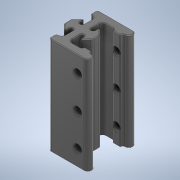
# Autodesk Inventor part: 80-20 Slider -  ( Length = 3 inch )
Saved by Autodesk Inventor 2020.2 (Build 242310000, 310)
## iProperties
Created: 2020-02-10
Part Number: 80-20 Slider -  ( Length = 3 inch )
Material: Generic
Document SubType Name: Modeling
Designer: lucas
Density: 1 g/cm^3
Appearance: Smooth - Black
Author: lucas
Autodesk Inventor part; units mm, degrees
ref_plane "YZ Plane" through (0, 0, 0) normal (1, 0, 0) x (0, 1, 0)
ref_plane "XZ Plane" through (0, 0, 0) normal (0, 1, 0) x (-1, 0, 0)
ref_plane "XY Plane" through (0, 0, 0) normal (0, 0, 1) x (1, 0, 0)
sketch "Sketch1" plane through (0, 0, 0) normal (0, 1, 0) x (-1, 0, 0)
  circle A0 centre (0, 0) radius 2.6035
  arc A1 (-12.6998, -10.5664) -> (-10.5664, -12.6998) centre (-10.5918, -10.5918) ccw
  arc A2 (-9.5504, -12.7) -> (-10.5664, -12.6998) centre (-10.0584, -12.7) ccw
  line L0 (-9.5504, -12.7) -> (-6.3331, -12.7)
  arc A3 (-5.3171, -12.7) -> (-6.3331, -12.7) centre (-5.8251, -12.7) ccw
  line L1 (-5.3171, -12.7) -> (-4.3434, -12.7)
  arc A4 (-4.3434, -12.7) -> (-4.3434, -10.4902) centre (-4.3434, -11.5951) ccw
  line L2 (-4.3434, -10.4902) -> (-6.4748, -10.4902)
  arc A5 (-7.1932, -8.7558) -> (-6.4748, -10.4902) centre (-6.4748, -9.4742) ccw
  line L3 (-7.1932, -8.7558) -> (-3.8632, -5.4257)
  arc A6 (-1.6181, -4.4958) -> (-3.8632, -5.4257) centre (-1.6181, -7.6708) ccw
  line L4 (-1.6181, -4.4958) -> (1.6181, -4.4958)
  arc A7 (3.8632, -5.4257) -> (1.6181, -4.4958) centre (1.6181, -7.6708) ccw
  line L5 (3.8632, -5.4257) -> (7.1932, -8.7558)
  arc A8 (6.4748, -10.4902) -> (7.1932, -8.7558) centre (6.4748, -9.4742) ccw
  line L6 (6.4748, -10.4902) -> (4.3434, -10.4902)
  arc A9 (4.3434, -10.4902) -> (4.3434, -12.7) centre (4.3434, -11.5951) ccw
  line L7 (4.3434, -12.7) -> (5.3171, -12.7)
  arc A10 (6.3331, -12.7) -> (5.3171, -12.7) centre (5.8251, -12.7) ccw
  line L8 (6.3331, -12.7) -> (9.5504, -12.7)
  arc A11 (10.5664, -12.6998) -> (9.5504, -12.7) centre (10.0584, -12.7) ccw
  arc A12 (10.5664, -12.6998) -> (12.6998, -10.5664) centre (10.5918, -10.5918) ccw
  arc A13 (12.7, -9.5504) -> (12.6998, -10.5664) centre (12.7, -10.0584) ccw
  line L9 (12.7, -9.5504) -> (12.7, -6.3331)
  arc A14 (12.7, -5.3171) -> (12.7, -6.3331) centre (12.7, -5.8251) ccw
  line L10 (12.7, -5.3171) -> (12.7, -4.3434)
  arc A15 (12.7, -4.3434) -> (10.4902, -4.3434) centre (11.5951, -4.3434) ccw
  line L11 (10.4902, -4.3434) -> (10.4902, -6.4748)
  arc A16 (8.7558, -7.1932) -> (10.4902, -6.4748) centre (9.4742, -6.4748) ccw
  line L12 (8.7558, -7.1932) -> (5.4257, -3.8632)
  arc A17 (4.4958, -1.6181) -> (5.4257, -3.8632) centre (7.6708, -1.6181) ccw
  line L13 (4.4958, -1.6181) -> (4.4958, 1.6181)
  arc A18 (5.4257, 3.8632) -> (4.4958, 1.6181) centre (7.6708, 1.6181) ccw
  line L14 (5.4257, 3.8632) -> (8.7558, 7.1932)
  arc A19 (10.4902, 6.4748) -> (8.7558, 7.1932) centre (9.4742, 6.4748) ccw
  line L15 (10.4902, 6.4748) -> (10.4902, 4.3434)
  arc A20 (10.4902, 4.3434) -> (12.7, 4.3434) centre (11.5951, 4.3434) ccw
  line L16 (12.7, 4.3434) -> (12.7, 5.3171)
  arc A21 (12.7, 6.3331) -> (12.7, 5.3171) centre (12.7, 5.8251) ccw
  line L17 (12.7, 6.3331) -> (12.7, 9.5504)
  arc A22 (12.6998, 10.5664) -> (12.7, 9.5504) centre (12.7, 10.0584) ccw
  arc A23 (12.6998, 10.5664) -> (10.5664, 12.6998) centre (10.5918, 10.5918) ccw
  arc A24 (9.5504, 12.7) -> (10.5664, 12.6998) centre (10.0584, 12.7) ccw
  line L18 (9.5504, 12.7) -> (6.3331, 12.7)
  arc A25 (5.3171, 12.7) -> (6.3331, 12.7) centre (5.8251, 12.7) ccw
  line L19 (5.3171, 12.7) -> (4.3434, 12.7)
  arc A26 (4.3434, 12.7) -> (4.3434, 10.4902) centre (4.3434, 11.5951) ccw
  line L20 (4.3434, 10.4902) -> (6.4748, 10.4902)
  arc A27 (7.1932, 8.7558) -> (6.4748, 10.4902) centre (6.4748, 9.4742) ccw
  line L21 (7.1932, 8.7558) -> (3.8632, 5.4257)
  arc A28 (1.6181, 4.4958) -> (3.8632, 5.4257) centre (1.6181, 7.6708) ccw
  line L22 (1.6181, 4.4958) -> (-1.6181, 4.4958)
  arc A29 (-3.8632, 5.4257) -> (-1.6181, 4.4958) centre (-1.6181, 7.6708) ccw
  line L23 (-3.8632, 5.4257) -> (-7.1932, 8.7558)
  arc A30 (-6.4748, 10.4902) -> (-7.1932, 8.7558) centre (-6.4748, 9.4742) ccw
  line L24 (-6.4748, 10.4902) -> (-4.3434, 10.4902)
  arc A31 (-4.3434, 10.4902) -> (-4.3434, 12.7) centre (-4.3434, 11.5951) ccw
  line L25 (-4.3434, 12.7) -> (-5.3171, 12.7)
  arc A32 (-6.3331, 12.7) -> (-5.3171, 12.7) centre (-5.8251, 12.7) ccw
  line L26 (-6.3331, 12.7) -> (-9.5504, 12.7)
  arc A33 (-10.5664, 12.6998) -> (-9.5504, 12.7) centre (-10.0584, 12.7) ccw
  arc A34 (-10.5664, 12.6998) -> (-12.6998, 10.5664) centre (-10.5918, 10.5918) ccw
  arc A35 (-12.7, 9.5504) -> (-12.6998, 10.5664) centre (-12.7, 10.0584) ccw
  line L27 (-12.7, 9.5504) -> (-12.7, 6.3331)
  arc A36 (-12.7, 5.3171) -> (-12.7, 6.3331) centre (-12.7, 5.8251) ccw
  line L28 (-12.7, 5.3171) -> (-12.7, 4.3434)
  arc A37 (-12.7, 4.3434) -> (-10.4902, 4.3434) centre (-11.5951, 4.3434) ccw
  line L29 (-10.4902, 4.3434) -> (-10.4902, 6.4748)
  arc A38 (-8.7558, 7.1932) -> (-10.4902, 6.4748) centre (-9.4742, 6.4748) ccw
  line L30 (-8.7558, 7.1932) -> (-5.4257, 3.8632)
  arc A39 (-4.4958, 1.6181) -> (-5.4257, 3.8632) centre (-7.6708, 1.6181) ccw
  line L31 (-4.4958, 1.6181) -> (-4.4958, -1.6181)
  arc A40 (-5.4257, -3.8632) -> (-4.4958, -1.6181) centre (-7.6708, -1.6181) ccw
  line L32 (-5.4257, -3.8632) -> (-8.7558, -7.1932)
  arc A41 (-10.4902, -6.4748) -> (-8.7558, -7.1932) centre (-9.4742, -6.4748) ccw
  line L33 (-10.4902, -6.4748) -> (-10.4902, -4.3434)
  arc A42 (-10.4902, -4.3434) -> (-12.7, -4.3434) centre (-11.5951, -4.3434) ccw
  line L34 (-12.7, -4.3434) -> (-12.7, -5.3171)
  arc A43 (-12.7, -6.3331) -> (-12.7, -5.3171) centre (-12.7, -5.8251) ccw
  line L35 (-12.7, -6.3331) -> (-12.7, -9.5504)
  arc A44 (-12.6998, -10.5664) -> (-12.7, -9.5504) centre (-12.7, -10.0584) ccw
  arc A45 (-10.1902, -6.4748) -> (-8.9679, -6.9811) centre (-9.4742, -6.4748) ccw
  arc A46 (-8.9679, 6.9811) -> (-10.1902, 6.4748) centre (-9.4742, 6.4748) ccw
  line L36 (-8.9679, 6.9811) -> (-5.6379, 3.651)
  arc A47 (-4.7958, 1.6181) -> (-5.6379, 3.651) centre (-7.6708, 1.6181) ccw
  arc A48 (-5.6379, -3.651) -> (-4.7958, -1.6181) centre (-7.6708, -1.6181) ccw
  line L37 (-4.7958, 1.6181) -> (-4.7958, -1.6181)
  line L38 (-5.6379, -3.651) -> (-8.9679, -6.9811)
  line L39 (-10.1902, 6.4748) -> (-10.1902, 4.3434)
  line L40 (-10.1902, -6.4748) -> (-10.1902, -4.3434)
  line L41 (-13.7, 19.05) -> (-39.37, 19.05)
  line L42 (-13, -4.3434) -> (-13, -10.5918)
  line L43 (-13.7, -19.05) -> (-39.37, -19.05)
  line L44 (-3.005, 15.2109) -> (-3.005, 14.9109)
  arc A49 (-13, 4.3434) -> (-10.1902, 4.3434) centre (-11.5951, 4.3434) ccw
  line L45 (-13, 4.3434) -> (-13, 10.5918)
  arc A50 (-10.1902, -4.3434) -> (-13, -4.3434) centre (-11.5951, -4.3434) ccw
  line L46 (-39.37, 19.05) -> (-39.37, -19.05)
  line L47 (-13.7, 19.05) -> (-8.89, 19.05)
  line L48 (-8.89, 19.05) -> (-8.89, 13)
  line L49 (-8.89, 13) -> (-10.5918, 13)
  line L50 (-13.7, -19.05) -> (-8.89, -19.05)
  line L51 (-8.89, -19.05) -> (-8.89, -13)
  line L52 (-8.89, -13) -> (-10.5918, -13)
  arc A51 (-10.5918, 13) -> (-13, 10.5918) centre (-10.5918, 10.5918) ccw
  arc A52 (-13, -10.5918) -> (-10.5918, -13) centre (-10.5918, -10.5918) ccw
  line L53 (-15.875, -23.3068) -> (-15.875, 30.5551) construction
  line L54 (-35.6132, -5.4257) -> (-38.9432, -8.7558)
  line L55 (-38.2248, -10.4902) -> (-36.0934, -10.4902)
  line L56 (-36.0934, -12.7) -> (-37.0671, -12.7)
  arc A53 (-36.0934, -12.7) -> (-36.0934, -10.4902) centre (-36.0934, -11.5951) ccw
  arc A54 (-37.1757, -3.8632) -> (-36.2458, -1.6181) centre (-39.4208, -1.6181) ccw
  arc A55 (-33.3681, -4.4958) -> (-35.6132, -5.4257) centre (-33.3681, -7.6708) ccw
  line L57 (-30.1319, -4.4958) -> (-33.3681, -4.4958)
  arc A56 (-37.0671, -12.7) -> (-38.0831, -12.7) centre (-37.5751, -12.7) ccw
  arc A57 (-36.2458, 1.6181) -> (-37.1757, 3.8632) centre (-39.4208, 1.6181) ccw
  line L58 (-36.2458, -1.6181) -> (-36.2458, 1.6181)
  arc A58 (-24.5568, 8.7558) -> (-25.2752, 10.4902) centre (-25.2752, 9.4742) ccw
  arc A59 (-19.0502, 10.5664) -> (-19.05, 9.5504) centre (-19.05, 10.0584) ccw
  arc A60 (-19.0502, 10.5664) -> (-21.1836, 12.6998) centre (-21.1582, 10.5918) ccw
  arc A61 (-22.1996, 12.7) -> (-21.1836, 12.6998) centre (-21.6916, 12.7) ccw
  line L59 (-25.2752, 10.4902) -> (-27.4066, 10.4902)
  line L60 (-25.4169, 12.7) -> (-22.1996, 12.7)
  arc A62 (-26.4329, 12.7) -> (-25.4169, 12.7) centre (-25.9249, 12.7) ccw
  arc A63 (-27.4066, 12.7) -> (-27.4066, 10.4902) centre (-27.4066, 11.5951) ccw
  line L61 (-27.4066, 12.7) -> (-26.4329, 12.7)
  arc A64 (-22.9942, -7.1932) -> (-21.2598, -6.4748) centre (-22.2758, -6.4748) ccw
  line L62 (-24.5568, -8.7558) -> (-27.8868, -5.4257)
  line L63 (-19.05, -6.3331) -> (-19.05, -9.5504)
  arc A65 (-25.2752, -10.4902) -> (-24.5568, -8.7558) centre (-25.2752, -9.4742) ccw
  arc A66 (-19.05, -9.5504) -> (-19.0502, -10.5664) centre (-19.05, -10.0584) ccw
  line L64 (-27.4066, -10.4902) -> (-25.2752, -10.4902)
  arc A67 (-21.1836, -12.6998) -> (-19.0502, -10.5664) centre (-21.1582, -10.5918) ccw
  arc A68 (-21.1836, -12.6998) -> (-22.1996, -12.7) centre (-21.6916, -12.7) ccw
  line L65 (-22.1996, -12.7) -> (-25.4169, -12.7)
  arc A69 (-25.4169, -12.7) -> (-26.4329, -12.7) centre (-25.9249, -12.7) ccw
  arc A70 (-27.4066, -10.4902) -> (-27.4066, -12.7) centre (-27.4066, -11.5951) ccw
  line L66 (-26.4329, -12.7) -> (-27.4066, -12.7)
  arc A71 (-38.9432, -8.7558) -> (-38.2248, -10.4902) centre (-38.2248, -9.4742) ccw
  line L67 (-40.5058, -7.1932) -> (-37.1757, -3.8632)
  line L68 (-38.0831, -12.7) -> (-41.3004, -12.7)
  arc A72 (-42.2402, -6.4748) -> (-40.5058, -7.1932) centre (-41.2242, -6.4748) ccw
  arc A73 (-41.3004, -12.7) -> (-42.3164, -12.6998) centre (-41.8084, -12.7) ccw
  line L69 (-42.2402, -4.3434) -> (-42.2402, -6.4748)
  arc A74 (-42.2402, -4.3434) -> (-44.45, -4.3434) centre (-43.3451, -4.3434) ccw
  line L70 (-44.45, -5.3171) -> (-44.45, -4.3434)
  arc A75 (-44.45, -6.3331) -> (-44.45, -5.3171) centre (-44.45, -5.8251) ccw
  line L71 (-44.45, -9.5504) -> (-44.45, -6.3331)
  arc A76 (-44.4498, -10.5664) -> (-44.45, -9.5504) centre (-44.45, -10.0584) ccw
  arc A77 (-44.4498, -10.5664) -> (-42.3164, -12.6998) centre (-42.3418, -10.5918) ccw
  line L72 (-37.1757, 3.8632) -> (-40.5058, 7.1932)
  line L73 (-42.2402, 6.4748) -> (-42.2402, 4.3434)
  arc A78 (-44.45, 4.3434) -> (-42.2402, 4.3434) centre (-43.3451, 4.3434) ccw
  line L74 (-38.9432, 8.7558) -> (-35.6132, 5.4257)
  line L75 (-44.45, 4.3434) -> (-44.45, 5.3171)
  arc A79 (-40.5058, 7.1932) -> (-42.2402, 6.4748) centre (-41.2242, 6.4748) ccw
  line L76 (-36.0934, 10.4902) -> (-38.2248, 10.4902)
  arc A80 (-44.45, 5.3171) -> (-44.45, 6.3331) centre (-44.45, 5.8251) ccw
  line L77 (-44.45, 6.3331) -> (-44.45, 9.5504)
  arc A81 (-44.45, 9.5504) -> (-44.4498, 10.5664) centre (-44.45, 10.0584) ccw
  arc A82 (-38.2248, 10.4902) -> (-38.9432, 8.7558) centre (-38.2248, 9.4742) ccw
  arc A83 (-36.0934, 10.4902) -> (-36.0934, 12.7) centre (-36.0934, 11.5951) ccw
  line L78 (-37.0671, 12.7) -> (-36.0934, 12.7)
  arc A84 (-38.0831, 12.7) -> (-37.0671, 12.7) centre (-37.5751, 12.7) ccw
  line L79 (-41.3004, 12.7) -> (-38.0831, 12.7)
  arc A85 (-42.3164, 12.6998) -> (-41.3004, 12.7) centre (-41.8084, 12.7) ccw
  arc A86 (-42.3164, 12.6998) -> (-44.4498, 10.5664) centre (-42.3418, 10.5918) ccw
  circle A87 centre (-31.75, 0) radius 2.6035
  arc A88 (-35.6132, 5.4257) -> (-33.3681, 4.4958) centre (-33.3681, 7.6708) ccw
  line L80 (-33.3681, 4.4958) -> (-30.1319, 4.4958)
  arc A89 (-30.1319, 4.4958) -> (-27.8868, 5.4257) centre (-30.1319, 7.6708) ccw
  line L81 (-19.05, 9.5504) -> (-19.05, 6.3331)
  line L82 (-27.8868, 5.4257) -> (-24.5568, 8.7558)
  arc A90 (-21.2598, 6.4748) -> (-22.9942, 7.1932) centre (-22.2758, 6.4748) ccw
  arc A91 (-19.05, 6.3331) -> (-19.05, 5.3171) centre (-19.05, 5.8251) ccw
  line L83 (-21.2598, 4.3434) -> (-21.2598, 6.4748)
  line L84 (-22.9942, 7.1932) -> (-26.3243, 3.8632)
  arc A92 (-26.3243, 3.8632) -> (-27.2542, 1.6181) centre (-24.0792, 1.6181) ccw
  line L85 (-19.05, 5.3171) -> (-19.05, 4.3434)
  arc A93 (-21.2598, 4.3434) -> (-19.05, 4.3434) centre (-20.1549, 4.3434) ccw
  arc A94 (-27.8868, -5.4257) -> (-30.1319, -4.4958) centre (-30.1319, -7.6708) ccw
  line L86 (-21.2598, -6.4748) -> (-21.2598, -4.3434)
  arc A95 (-19.05, -5.3171) -> (-19.05, -6.3331) centre (-19.05, -5.8251) ccw
  line L87 (-19.05, -4.3434) -> (-19.05, -5.3171)
  arc A96 (-19.05, -4.3434) -> (-21.2598, -4.3434) centre (-20.1549, -4.3434) ccw
  arc A97 (-27.2542, -1.6181) -> (-26.3243, -3.8632) centre (-24.0792, -1.6181) ccw
  line L88 (-27.2542, 1.6181) -> (-27.2542, -1.6181)
  line L89 (-26.3243, -3.8632) -> (-22.9942, -7.1932)
  arc A98 (-21.5598, 6.4748) -> (-22.7821, 6.9811) centre (-22.2758, 6.4748) ccw
  line L90 (-22.7821, 6.9811) -> (-26.1121, 3.651)
  arc A99 (-26.1121, 3.651) -> (-26.9542, 1.6181) centre (-24.0792, 1.6181) ccw
  line L91 (-26.9542, 1.6181) -> (-26.9542, -1.6181)
  arc A100 (-26.9542, -1.6181) -> (-26.1121, -3.651) centre (-24.0792, -1.6181) ccw
  line L92 (-26.1121, -3.651) -> (-22.7821, -6.9811)
  arc A101 (-22.7821, -6.9811) -> (-21.5598, -6.4748) centre (-22.2758, -6.4748) ccw
  line L93 (-21.5598, 6.4748) -> (-21.5598, 4.3434)
  line L94 (-21.5598, -6.4748) -> (-21.5598, -4.3434)
  line L95 (-18.75, -4.3434) -> (-18.75, -10.5918)
  arc A102 (-21.5598, 4.3434) -> (-18.75, 4.3434) centre (-20.1549, 4.3434) ccw
  line L96 (-18.75, 4.3434) -> (-18.75, 10.5918)
  arc A103 (-18.75, -4.3434) -> (-21.5598, -4.3434) centre (-20.1549, -4.3434) ccw
  arc A104 (-18.75, 10.5918) -> (-21.1582, 13) centre (-21.1582, 10.5918) ccw
  arc A105 (-21.1582, -13) -> (-18.75, -10.5918) centre (-21.1582, -10.5918) ccw
  arc A106 (-24.7689, 8.9679) -> (-25.2752, 10.1902) centre (-25.2752, 9.4742) ccw
  line L97 (-25.2752, 10.1902) -> (-27.4066, 10.1902)
  arc A107 (-35.401, 5.6379) -> (-33.3681, 4.7958) centre (-33.3681, 7.6708) ccw
  line L98 (-33.3681, 4.7958) -> (-30.1319, 4.7958)
  arc A108 (-30.1319, 4.7958) -> (-28.099, 5.6379) centre (-30.1319, 7.6708) ccw
  line L99 (-28.099, 5.6379) -> (-24.7689, 8.9679)
  line L100 (-38.7311, 8.9679) -> (-35.401, 5.6379)
  line L101 (-38.2248, 10.1902) -> (-36.0934, 10.1902)
  arc A109 (-36.0934, 10.1902) -> (-36.0934, 13) centre (-36.0934, 11.5951) ccw
  arc A110 (-27.4066, 13) -> (-27.4066, 10.1902) centre (-27.4066, 11.5951) ccw
  arc A111 (-38.2248, 10.1902) -> (-38.7311, 8.9679) centre (-38.2248, 9.4742) ccw
  arc A112 (-40.7179, 6.9811) -> (-41.9402, 6.4748) centre (-41.2242, 6.4748) ccw
  line L102 (-41.9402, 6.4748) -> (-41.9402, 4.3434)
  arc A113 (-37.3879, -3.651) -> (-36.5458, -1.6181) centre (-39.4208, -1.6181) ccw
  line L103 (-36.5458, -1.6181) -> (-36.5458, 1.6181)
  arc A114 (-36.5458, 1.6181) -> (-37.3879, 3.651) centre (-39.4208, 1.6181) ccw
  line L104 (-37.3879, 3.651) -> (-40.7179, 6.9811)
  line L105 (-40.7179, -6.9811) -> (-37.3879, -3.651)
  line L106 (-41.9402, -6.4748) -> (-41.9402, -4.3434)
  arc A115 (-41.9402, -4.3434) -> (-44.75, -4.3434) centre (-43.3451, -4.3434) ccw
  arc A116 (-44.75, 4.3434) -> (-41.9402, 4.3434) centre (-43.3451, 4.3434) ccw
  arc A117 (-41.9402, -6.4748) -> (-40.7179, -6.9811) centre (-41.2242, -6.4748) ccw
  arc A118 (-38.7311, -8.9679) -> (-38.2248, -10.1902) centre (-38.2248, -9.4742) ccw
  line L107 (-38.2248, -10.1902) -> (-36.0934, -10.1902)
  arc A119 (-28.099, -5.6379) -> (-30.1319, -4.7958) centre (-30.1319, -7.6708) ccw
  line L108 (-30.1319, -4.7958) -> (-33.3681, -4.7958)
  arc A120 (-33.3681, -4.7958) -> (-35.401, -5.6379) centre (-33.3681, -7.6708) ccw
  line L109 (-35.401, -5.6379) -> (-38.7311, -8.9679)
  line L110 (-24.7689, -8.9679) -> (-28.099, -5.6379)
  line L111 (-25.2752, -10.1902) -> (-27.4066, -10.1902)
  arc A121 (-27.4066, -10.1902) -> (-27.4066, -13) centre (-27.4066, -11.5951) ccw
  arc A122 (-36.0934, -13) -> (-36.0934, -10.1902) centre (-36.0934, -11.5951) ccw
  arc A123 (-25.2752, -10.1902) -> (-24.7689, -8.9679) centre (-25.2752, -9.4742) ccw
  line L112 (-21.1582, -13) -> (-27.4066, -13)
  line L113 (-36.0934, -13) -> (-39.37, -13)
  line L114 (-27.4066, 13) -> (-21.1582, 13)
  line L115 (-36.0934, 13) -> (-39.37, 13)
  dimension "d0" = 0.3
  dimension "d1" = 0.3
  dimension "d4" = 0.3
  dimension "d5" = 0.3
  dimension "d10" = 3.2362
  dimension "d13" = 6.35
  dimension "d14" = 6.35
  dimension "d15" = 0.3
  dimension "d17" = 0.3
  dimension "d22" = 0.3
  dimension "d24" = 3.81
  dimension "d25" = 15.875
  dimension "d26" = 5.08
  dimension "d29" = 360
  dimension "d62" = 0.3
  dimension "d63" = 0.3
  dimension "d64" = 0.3
  constraints: 244 point on circle, 232 end point, 155 symmetric about line, 124 centre point, 20 vertical, 17 horizontal, 14 tangent, 4 concentric, 4 point on line, 3 parallel, 3 perpendicular, 2 collinear, 1 vertical alignment, 349 other
  measures "d0" distance between parallel lines of L31 L37
  measures "d1" distance between parallel lines of L30 L36
  measures "d4" distance between parallel lines of L32 L38
  measures "d5" distance between parallel lines of L29 L39
  measures "d10" distance of A40.centre A39.centre
  measures "d13" distance between parallel lines of L26 L41
  measures "d14" distance between parallel lines of L0 L43
  measures "d15" distance between parallel lines of L35 L42
  measures "d17" distance of L44.start L44.end
  measures "d22" distance between parallel lines of L0 L52
  measures "d24" distance between parallel lines of L27 L48
  measures "d25" distance from line of L53 point (0, 0)
  measures "d26" distance between parallel lines of L77 L46
  measures "d62" radial gap between concentric circles of A38 A46
  measures "d63" radial gap between concentric circles of A41 A45
  measures "d64" radial gap between concentric circles of A39 A47
extrude "Extrusion1" add sketch "Sketch1" along normal blind 76.2 contours L40 A50 L42 A52 L52 L51 L50 L43 L46 L113 A122 L107 A118 L109 A120 L108 A119 L110 A123 L111 A121 L112 A105 L95 A103 L94 A101 L92 A100 L91 A99 L90 A98 L93 A102 L96 A104 L114 A110 L97 A106 L99 A108 L98 A107 L100 A111 L101 A109 L115 L41 L47 L48 L49 A51 L45 A49 L39 A46 L36 A47 L37 A48 L38 A45
full round fillet "Fillet3" first side at (22.2567, 50.8, 19.05) centre faces at (39.37, 25.4, 17.0333) second side at (38.2778, 25.4, 13)
full round fillet "Fillet4" first side at (37.1856, 25.4, -13) centre faces at (39.37, 25.4, -15.0167) second side at (30.8133, 25.4, -19.05)
sketch "Sketch2" plane through (0, 76.2, 0) normal (0, 1, 0) x (1, 0, 0)
  line L0 (22.2176, -11) -> (42.7005, -11)
  line L1 (42.7005, -11) -> (42.7005, 11)
  line L2 (42.7005, 11) -> (22.2176, 11)
  line L3 (22.2176, 11) -> (22.2176, -11)
  line L4 (21.9249, 0) -> (54.1946, 0)
  line L5 (27.4066, -13) -> (21.1582, -13) projected
  line L6 (36.345, 19.05) -> (8.89, 19.05) projected
  line L7 (8.89, -19.05) -> (36.345, -19.05) projected
  line L8 (33.3681, -4.7958) -> (30.1319, -4.7958) projected
  line L9 (26.9542, -1.6181) -> (26.9542, 1.6181) projected
  line L10 (30.1319, 4.7958) -> (33.3681, 4.7958) projected
  line L11 (22.2176, 7.6919) -> (30.2043, -0.3698)
  line L12 (30.2043, -0.3698) -> (22.2176, -8.2822)
  line L13 (27.4066, 10.1902) -> (25.2752, 10.1902) projected
  line L14 (25.2752, -10.1902) -> (27.4066, -10.1902) projected
  line L15 (21.1582, 13) -> (27.4066, 13) projected
  point P0 (0, 0)
  point P1 (10.295, 16.51)
  point P2 (10.295, -16.51)
  point P3 (8.89, 19.05)
  point P4 (23.2231, 10.9)
  point P5 (15.6239, 0)
  dimension "d35" = 38.1
  dimension "d36" = 19.05
  dimension "d78" = 19.05
  dimension "d81" = 2
  dimension "d82" = 2
  constraints: 14 end point, 2 horizontal, 2 parallel, 2 perpendicular, 2 point on line, 2 other
  measures "d81" distance between parallel lines of L15 L2
  measures "d82" distance between parallel lines of L5 L0
extrude "Extrusion2" cut sketch "Sketch2" against normal through all contours L3 L12 L11 L4 L1 L0 | L4 L11 L3 L2 L1
fillet "Fillet7" radius 0.508 4 edges at (34.8208, 38.1, 11) (28.6792, 38.1, 11) (28.6792, 38.1, -11) (34.8208, 38.1, -11)
fillet "Fillet8" radius 2.032 4 edges at (8.89, 38.1, 19.05) (8.89, 38.1, 13) (8.89, 38.1, -13) (8.89, 38.1, -19.05)
sketch "Sketch4" plane through (36.345, 0, 19.05) normal (0, 0, 1) x (1, 0, 0)
  line L0 (-2.1625, 76.2) -> (-2.1625, 0) construction
  line L1 (-7.0275, 76.2) -> (-2.1625, 76.2) projected
  line L2 (-7.0275, 0) -> (-7.0275, 76.2) construction
  line L3 (-2.1625, 0) -> (-7.0275, 0) projected
  circle A0 centre (-4.8776, 38.1) radius 3.175
  circle A1 centre (-4.8776, 63.5) radius 3.175
  circle A2 centre (-4.8776, 12.7) radius 3.175
  point P0 (-36.345, 0)
  dimension "d67" = 76.2
  dimension "d68" = 38.1
  dimension "d69" = 25.4
  dimension "d70" = 25.4
  dimension "d71" = 6.35
  constraints: 3 centre point, 2 equal radius
  measures "d67" distance of L0.start L0.end
  measures "d68" vertical distance of A0.centre L0.start
  measures "d69" distance of A0.centre A1.centre
  measures "d70" distance of A2.centre A0.centre
  measures "d71" diameter of A0
extrude "Extrusion4" cut sketch "Sketch4" against normal through all
chamfer "Chamfer2" distance 0.508 angle 45 112 edges at (23.6335, 76.2, 19.05) (38.484, 76.2, 18.164) (38.484, 76.2, 13.886) (36.2192, 76.2, 13) (35.0776, 76.2, 12.5656) (34.5498, 76.2, 11.1571) (31.75, 76.2, 11) (28.9502, 76.2, 11.1571) (28.4224, 76.2, 12.5656) (24.2824, 76.2, 13) (19.4553, 76.2, 12.2947) (18.75, 76.2, 7.4676) (20.1549, 76.2, 2.9385) (21.5598, 76.2, 5.4091) (22.0018, 76.2, 7.1363) (24.4471, 76.2, 5.3161) (26.7354, 76.2, 2.7183) (26.9542, 76.2, 0) (26.7354, 76.2, -2.7183) (24.4471, 76.2, -5.3161) (22.0018, 76.2, -7.1363) (21.5598, 76.2, -5.4091) (20.1549, 76.2, -2.9385) (18.75, 76.2, -7.4676) (19.4553, 76.2, -12.2947) (24.2824, 76.2, -13) (28.4224, 76.2, -12.5656) (28.9502, 76.2, -11.1571) (31.75, 76.2, -11) (34.5498, 76.2, -11.1571) (35.0776, 76.2, -12.5656) (36.2192, 76.2, -13) (38.484, 76.2, -18.164) (38.484, 76.2, -13.886) (23.6335, 76.2, -19.05) (9.4852, 76.2, -18.4548) (8.89, 76.2, -16.0189) (9.4327, 76.2, -13.6373) (12.3568, 76.2, -12.2301) (13, 76.2, -7.4676) (11.5951, 76.2, -2.9385) (10.1902, 76.2, -5.4091) (9.7482, 76.2, -7.1363) (7.3029, 76.2, -5.3161) (5.0146, 76.2, -2.7183) (4.7958, 76.2, 0) (5.0146, 76.2, 2.7183) (7.3029, 76.2, 5.3161) (9.7482, 76.2, 7.1363) (10.1902, 76.2, 5.4091) (11.5951, 76.2, 2.9385) (13, 76.2, 7.4676) (12.3568, 76.2, 12.2301) (9.4327, 76.2, 13.6373) (8.89, 76.2, 16.0189) (9.4852, 76.2, 18.4548) (23.6335, 0, 19.05) (38.484, 0, 18.164) (38.484, 0, 13.886) (36.2192, 0, 13) (35.0776, 0, 12.5656) (34.5498, 0, 11.1571) (31.75, 0, 11) (28.9502, 0, 11.1571) (28.4224, 0, 12.5656) (24.2824, 0, 13) (19.4553, 0, 12.2947) (18.75, 0, 7.4676) (20.1549, 0, 2.9385) (21.5598, 0, 5.4091) (22.0018, 0, 7.1363) (24.4471, 0, 5.3161) (26.7354, 0, 2.7183) (26.9542, 0, 0) (26.7354, 0, -2.7183) (24.4471, 0, -5.3161) (22.0018, 0, -7.1363) (21.5598, 0, -5.4091) (20.1549, 0, -2.9385) (18.75, 0, -7.4676) (19.4553, 0, -12.2947) (24.2824, 0, -13) (28.4224, 0, -12.5656) (28.9502, 0, -11.1571) (31.75, 0, -11) (34.5498, 0, -11.1571) (35.0776, 0, -12.5656) (36.2192, 0, -13) (38.484, 0, -18.164) (38.484, 0, -13.886) (23.6335, 0, -19.05) (9.4852, 0, -18.4548) (8.89, 0, -16.0189) (9.4327, 0, -13.6373) (12.3568, 0, -12.2301) (13, 0, -7.4676) (11.5951, 0, -2.9385) (10.1902, 0, -5.4091) (9.7482, 0, -7.1363) (7.3029, 0, -5.3161) (5.0146, 0, -2.7183) (4.7958, 0, 0) (5.0146, 0, 2.7183) (7.3029, 0, 5.3161) (9.7482, 0, 7.1363) (10.1902, 0, 5.4091) (11.5951, 0, 2.9385) (13, 0, 7.4676) (12.3568, 0, 12.2301) (9.4327, 0, 13.6373) (8.89, 0, 16.0189) (9.4852, 0, 18.4548)
equation "\"d1\" = d17"
equation "\"d4\" = d17"
equation "\"d5\" = d17"
equation "\"d14\" = d13"
equation "\"d15\" = d17"
equation "\"d22\" = d17"
equation "\"d36\" = 0.5 * d35"
body "Solid1"
